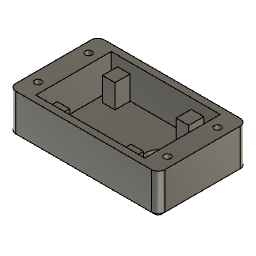
ThermaQR+-+camera+housing+main (Autodesk Fusion 360 design; units mm, degrees)
Autodesk Fusion 360 part; units mm, degrees
sketch "Sketch1" plane through (0, 0, 0) normal (0, 0, 1) x (1, 0, 0)
  line L0 (-16.25, 11.25) -> (16.25, 11.25)
  line L1 (16.25, 11.25) -> (16.25, -11.25)
  line L2 (16.25, -11.25) -> (-16.25, -11.25)
  line L3 (-16.25, -11.25) -> (-16.25, 11.25)
  line L4 (-22.25, 13.25) -> (22.25, 13.25)
  line L5 (22.25, 13.25) -> (22.25, -13.25)
  line L6 (22.25, -13.25) -> (-22.25, -13.25)
  line L7 (-22.25, -13.25) -> (-22.25, 13.25)
  line L8 (-22.25, 13.25) -> (22.25, -13.25) construction
  line L9 (22.25, 13.25) -> (-22.25, -13.25) construction
  line L10 (-19.25, 7.5) -> (-19.25, -7.5) construction
  line L11 (-22.25, 0) -> (-16.25, 0) construction
  line L12 (16.25, 0) -> (22.25, 0) construction
  line L13 (19.25, 7.5) -> (19.25, -7.5) construction
  circle A0 centre (-19.25, 7.5) radius 1
  circle A1 centre (-19.25, -7.5) radius 1
  circle A2 centre (19.25, -7.5) radius 1
  circle A3 centre (19.25, 7.5) radius 1
  point P0 (-19.25, 0)
  point P1 (-19.25, 0)
  point P2 (19.25, 0)
  point P3 (19.25, 0)
  dimension "d1" = 32.5
  dimension "d2" = 22.5
  dimension "d3" = 2
  dimension "d4" = 6
  dimension "d21" = 6
  dimension "d22" = 2
  dimension "d23" = 15
  dimension "d24" = 2
  constraint horizontal L0
  constraint perpendicular L0 L1
  constraint parallel L0 L2
  constraint parallel L1 L3
  constraint horizontal L4
  constraint perpendicular L4 L5
  constraint parallel L4 L6
  constraint parallel L5 L7
  constraint coincident L8 origin
  constraint coincident L9 origin
  constraint vertical L10
  constraint midpoint L7 L11.start
  constraint midpoint L3 L11.end
  constraint midpoint L11 P1
  constraint midpoint L10 P1
  constraint coincident P1 P0
  constraint midpoint L1 L12.start
  constraint midpoint L5 L12.end
  constraint parallel L1 L13
  constraint midpoint L13 P3
  constraint midpoint L12 P3
  constraint coincident P3 P2
  constraint equal L10 L13
  constraint coincident L10.start A0.centre
  constraint coincident L10.end A1.centre
  constraint coincident L13.end A2.centre
  constraint coincident L13.start A3.centre
  constraint equal A1 A2
  constraint equal A2 A3
  constraint equal A0 A3
  measures "d1" distance of L0.start L0.end
  measures "d2" distance of L0.start L2.end
  measures "d3" distance of L0 L4
  measures "d4" distance of L1 L5
  measures "d21" distance of L3 L7
  measures "d22" distance of L2 L6
  measures "d23" distance of L10.start L10.end
  measures "d24" diameter of A0
extrude "Extrude1" add sketch "Sketch1" against normal blind 2 contours L0 L1 L2 L3 | L4 L5 L6 L7
extrude "Extrude2" add sketch "Sketch1" along normal blind 10
sketch "Sketch2" plane through (0, 0, 0) normal (0, 0, 1) x (-1, 0, 0)
  line L0 (-16.25, 11.25) -> (-16.25, -11.25)
  line L1 (-16.25, -11.25) -> (16.25, -11.25)
  line L2 (16.25, -11.25) -> (16.25, 11.25)
  line L3 (16.25, 11.25) -> (-16.25, 11.25)
  line L4 (12.5, 9) -> (12.5, -9) construction
  line L5 (12.5, -9) -> (-9.5, -9) construction
  line L6 (-9.5, 9) -> (12.5, 9) construction
  line L7 (-9.5, -9) -> (-9.5, 9) construction
  line L8 (12.5, -9) -> (-9.5, 9) construction
  line L9 (12.5, 9) -> (-9.5, -9) construction
  line L10 (14.375, -11.25) -> (10.625, -11.25)
  line L11 (10.625, -11.25) -> (10.625, -6.75)
  line L12 (10.625, -6.75) -> (14.375, -6.75)
  line L13 (14.375, -6.75) -> (14.375, -11.25)
  line L14 (14.375, -11.25) -> (10.625, -6.75) construction
  line L15 (10.625, -11.25) -> (14.375, -6.75) construction
  line L16 (-7.625, -11.25) -> (-11.375, -11.25)
  line L17 (-11.375, -11.25) -> (-11.375, -6.75)
  line L18 (-11.375, -6.75) -> (-7.625, -6.75)
  line L19 (-7.625, -6.75) -> (-7.625, -11.25)
  line L20 (-7.625, -11.25) -> (-11.375, -6.75) construction
  line L21 (-11.375, -11.25) -> (-7.625, -6.75) construction
  line L22 (14.375, 11.25) -> (10.625, 11.25)
  line L23 (10.625, 11.25) -> (10.625, 6.75)
  line L24 (10.625, 6.75) -> (14.375, 6.75)
  line L25 (14.375, 6.75) -> (14.375, 11.25)
  line L26 (14.375, 11.25) -> (10.625, 6.75) construction
  line L27 (10.625, 11.25) -> (14.375, 6.75) construction
  line L28 (-11.375, 11.25) -> (-7.625, 11.25)
  line L29 (-7.625, 11.25) -> (-7.625, 6.75)
  line L30 (-7.625, 6.75) -> (-11.375, 6.75)
  line L31 (-11.375, 6.75) -> (-11.375, 11.25)
  line L32 (-11.375, 11.25) -> (-7.625, 6.75) construction
  line L33 (-7.625, 11.25) -> (-11.375, 6.75) construction
  circle A0 centre (12.5, -9) radius 0.875
  circle A1 centre (-9.5, -9) radius 0.875
  circle A2 centre (-9.5, 9) radius 0.875
  circle A3 centre (12.5, 9) radius 0.875
  circle A4 centre (-9.5, 0) radius 4.5
  point P0 (1.5, 0)
  point P1 (12.5, -9)
  point P2 (-9.5, -9)
  point P3 (12.5, 9)
  point P4 (-9.5, 9)
  dimension "d9" = 18
  dimension "d10" = 22
  dimension "d11" = 1.5
  dimension "d12" = 3.75
  dimension "d13" = 1.75
  dimension "d16" = 9
  constraint perpendicular L4 L5
  constraint parallel L4 L7
  constraint parallel L5 L6
  constraint horizontal L5
  constraint midpoint L9 P0
  constraint horizontal origin P0
  constraint horizontal L10
  constraint perpendicular L10 L11
  constraint parallel L10 L12
  constraint parallel L11 L13
  constraint coincident L14 P1
  constraint coincident L15 P1
  constraint coincident L1 L10.start
  constraint coincident P1 L4.end
  constraint horizontal L16
  constraint perpendicular L16 L17
  constraint parallel L16 L18
  constraint parallel L17 L19
  constraint coincident L20 P2
  constraint coincident L21 P2
  constraint coincident L1 L16.start
  constraint coincident P2 L5.end
  constraint equal L12 L18
  constraint horizontal L22
  constraint perpendicular L22 L23
  constraint parallel L22 L24
  constraint parallel L23 L25
  constraint coincident L26 P3
  constraint coincident L27 P3
  constraint coincident L3 L22.start
  constraint coincident P3 L4.start
  constraint horizontal L28
  constraint perpendicular L28 L29
  constraint parallel L28 L30
  constraint parallel L29 L31
  constraint coincident L32 P4
  constraint coincident L33 P4
  constraint coincident P4 L6.start
  constraint equal L12 L24
  constraint equal L12 L30
  constraint coincident L3 L28.start
  constraint equal A2 A3
  constraint equal A1 A2
  constraint equal A0 A1
  constraint midpoint L7 A4.centre
  measures "d9" distance of P3 P1
  measures "d10" distance of P1 P2
  measures "d11" distance of origin P0
  measures "d12" distance of L11.end L12.end
  measures "d13" diameter of A0
  measures "d16" diameter of A4
extrude "Extrude3" add sketch "Sketch2" along normal blind 7 contours L3 L28 L29 L30 L31 | L1 L16 L17 L18 L19 | L3 L22 L23 L24 L25 | L1 L10 L11 L12 L13 | A0 | A1 | A2 | A3
extrude "Extrude4" cut sketch "Sketch2" against normal through all contours A4
sketch "Sketch3" plane through (0, 0, -2) normal (0, 0, -1) x (1, 0, 0)
  circle A0 centre (9.5, 0) radius 4.5
  circle A1 centre (19.25, -7.5) radius 1
  circle A2 centre (-19.25, 7.5) radius 1
  circle A3 centre (19.25, 7.5) radius 1
  circle A4 centre (-19.25, -7.5) radius 1
  line L0 (22.25, 13.25) -> (-22.25, 13.25)
  line L1 (-22.25, 13.25) -> (-22.25, -13.25)
  line L2 (-22.25, -13.25) -> (22.25, -13.25)
  line L3 (22.25, -13.25) -> (22.25, 13.25)
  circle A5 centre (-19.25, 7.5) radius 2
  circle A6 centre (-19.25, -7.5) radius 2
  circle A7 centre (19.25, -7.5) radius 2
  circle A8 centre (19.25, 7.5) radius 2
  dimension "d25" = 4
  constraint concentric A2 A5
  constraint concentric A4 A6
  constraint concentric A1 A7
  constraint concentric A3 A8
  constraint equal A5 A8
  constraint equal A7 A8
  constraint equal A6 A7
  measures "d25" diameter of A5
extrude "Extrude5" cut sketch "Sketch3" against normal blind 4 contours A5 | A6 | A7 | A8
fillet "Fillet1" radius 2 4 edges at (22.25, 13.25, 4) (-22.25, 13.25, 4) (-22.25, -13.25, 4) (22.25, -13.25, 4)
chamfer "Chamfer1" distance 1 angle 45 8 edges at (0, -13.25, -2) (-21.6642, -12.6642, -2) (-22.25, 0, -2) (-21.6642, 12.6642, -2) (0, 13.25, -2) (21.6642, 12.6642, -2) (22.25, 0, -2) (21.6642, -12.6642, -2)
equation "d21 = d4"
equation "d22 = d3"
